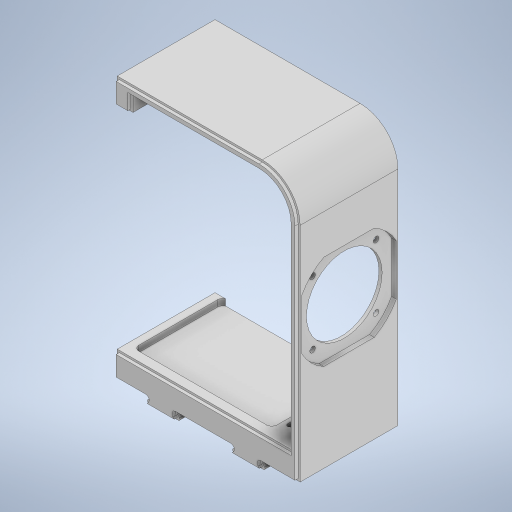
# Autodesk Inventor part: ElecTweetBox
Saved by Autodesk Inventor 2023 (Build 270158000, 158)
## iProperties
Created: 2022-07-12
Part Number: ElecTweetBox
Material: Generic
Document SubType Name: Modeling
Designer: Fuzzyfish
Density: 1 g/cm^3
Appearance: Default
Author: Fuzzyfish
Autodesk Inventor part; units mm, degrees
ref_plane "YZ Plane" through (0, 0, 0) normal (1, 0, 0) x (0, 1, 0)
ref_plane "XZ Plane" through (0, 0, 0) normal (0, 1, 0) x (-1, 0, 0)
ref_plane "XY Plane" through (0, 0, 0) normal (0, 0, 1) x (1, 0, 0)
sketch "Sketch1" plane through (0, 0, 0) normal (0, 0, 1) x (1, 0, 0)
  line L0 (0, 0) -> (116, 0)
  line L1 (116, 0) -> (116, 141)
  arc A0 (116, 141) -> (92, 165) centre (92, 141) ccw
  line L2 (0, 0) -> (0, 165)
  line L3 (0, 165) -> (92, 165)
  dimension "d0" = 24
  dimension "d1" = 92
  dimension "d2" = 165
  constraints: 8 end point, 2 horizontal, 2 point on circle, 2 tangent, 1 centre point, 1 perpendicular, 1 vertical
  measures "d0" radius of A0
  measures "d1" distance of L2.end L3.end
  measures "d2" distance of L0.start L2.end
extrude "Extrusion1" add sketch "Sketch1" along normal blind 62
shell "Shell2" thickness 5 removed faces 3 at (0, 110, 20.6667) at (38.6667, 102, 0) at (38.6667, 102, 62)
sketch "Sketch6" plane through (0, 160, 0) normal (0, -1, 0) x (1, 0, 0)
  line L0 (0, 0) -> (10, 0)
  line L1 (10, 0) -> (10, 10)
  line L2 (10, 10) -> (0, 10)
  line L3 (0, 10) -> (0, 0)
  dimension "d90" = 2
  dimension "d91" = 0
  dimension "d38" = 10
  dimension "d39" = 10
  constraints: 8 end point, 2 parallel, 1 horizontal, 1 perpendicular
  measures "d38" distance of L1.end L2.end
  measures "d39" distance of L0.end L1.end
sketch "Sketch7" plane through (0, 160, 0) normal (0, -1, 0) x (1, 0, 0)
  line L0 (0, 62) -> (10, 62)
  line L1 (10, 62) -> (10, 52)
  line L2 (10, 52) -> (0, 52)
  line L3 (0, 52) -> (0, 62)
  line L4 (92, 0) -> (0, 0) projected
  line L5 (92, 0) -> (92, 62) projected
  line L6 (0, 62) -> (92, 62) projected
  line L7 (0, 0) -> (0, 62) projected
  point P0 (0, 0)
  dimension "d40" = 10
  dimension "d41" = 10
  constraints: 8 end point, 2 parallel, 1 horizontal, 1 perpendicular
  measures "d40" distance of L1.end L2.end
  measures "d41" distance of L0.end L1.end
extrude "Extrusion6" add sketch "Sketch6" along normal blind 10
extrude "Extrusion7" add sketch "Sketch7" along normal blind 10 contours L0 L1 L2 L3
sketch "Sketch9" plane through (0, 5, 0) normal (0, 1, 0) x (1, 0, 0)
  line L0 (0, 0) -> (111, 0) projected
  line L1 (0, -62) -> (0, 0) projected
  line L2 (111, -62) -> (0, -62) projected
  line L3 (111, 0) -> (111, -62) projected
extrude "Extrusion8" add sketch "Sketch9" along normal blind 10
sketch "Sketch10" plane through (0, 15, 0) normal (0, 1, 0) x (1, 0, 0)
  arc A0 (5, -53) -> (8, -56) centre (8, -53) ccw
  arc A1 (8, 0) -> (5, -3) centre (8, -3) ccw
  line L0 (5, -53) -> (5, -3)
  arc A2 (92, -3) -> (89, 0) centre (89, -3) ccw
  arc A3 (89, -56) -> (92, -53) centre (89, -53) ccw
  line L1 (89, -56) -> (8, -56)
  line L2 (89, 0) -> (8, 0)
  line L3 (92, -53) -> (92, -3)
  line L4 (0, 0) -> (0, -62) projected
  line L5 (111, 0) -> (0, 0) projected
  arc A4 (4.7, -53) -> (8, -56.3) centre (8, -53) ccw
  line L6 (4.7, -53) -> (4.7, -3)
  arc A5 (8, 0.3) -> (4.7, -3) centre (8, -3) ccw
  line L7 (8, 0.3) -> (89, 0.3)
  arc A6 (92.3, -3) -> (89, 0.3) centre (89, -3) ccw
  line L8 (92.3, -3) -> (92.3, -53)
  arc A7 (89, -56.3) -> (92.3, -53) centre (89, -53) ccw
  line L9 (89, -56.3) -> (8, -56.3)
  point P0 (6.6252, 0)
  point P1 (90.3748, 0)
  point P2 (89, 0)
  dimension "d48" = 81
  dimension "d49" = 3
  dimension "d50" = 50
  dimension "d51" = 3
  dimension "d52" = 81
  dimension "d53" = 3
  dimension "d54" = 50
  dimension "d55" = 3
  dimension "d56" = 5
  dimension "d57" = 0.3
  constraints: 16 end point, 16 point on circle, 8 centre point, 6 tangent, 2 horizontal, 1 collinear, 1 vertical, 7 other
  measures "d48" distance of L1.start L1.end
  measures "d49" radius of A0
  measures "d50" distance of L0.start L0.end
  measures "d51" radius of A1
  measures "d52" distance of L2.start L2.end
  measures "d53" radius of A2
  measures "d54" distance of L3.start L3.end
  measures "d55" radius of A3
  measures "d56" distance between parallel lines of L0 L4
  measures "d57" distance between parallel lines of L9 L1
extrude "Extrusion9" cut sketch "Sketch10" against normal blind 4 contours L0 A1 L2 A2 L3 A3 L1 A0 | A0 L1 A3 L3 A2 L5 A6 L8 A7 L9 A4 L6 A5 A1 L0
sketch "Sketch12" plane through (0, 160, 10) normal (0, 0, 1) x (1, 0, 0)
  line L0 (0, 0) -> (10, 0) projected
  line L1 (0, 0) -> (0, -10) projected
  line L2 (10, -10) -> (0, -10) projected
  line L3 (10, 0) -> (10, -10) projected
  point P0 (0, -160)
extrude "Extrusion11" add sketch "Sketch12" along normal up to surface (42 mm away)
sketch "Sketch14" plane through (0, 0, 62) normal (0, 0, 1) x (1, 0, 0)
  line L0 (36.5757, 0) -> (41.5757, -5)
  line L1 (22, 0) -> (37, 0)
  line L2 (17.3, -4.7) -> (41.7, -4.7)
  line L3 (22.4243, 0) -> (17.4243, -5)
  line L4 (22, 0) -> (17, -5)
  line L5 (-3, 0) -> (-3, -5)
  line L6 (96, -5) -> (91, 0)
  line L7 (42, -5) -> (37, 0)
  line L8 (71, -5) -> (76, 0)
  line L9 (76.4243, 0) -> (71.4243, -5)
  line L10 (76, 0) -> (91, 0)
  line L11 (71.3, -4.7) -> (95.7, -4.7)
  line L12 (116, 0) -> (-3, 0)
  line L13 (-3, 0) -> (116, 0)
  line L14 (-3, -5) -> (116, -5)
  line L15 (90.5757, 0) -> (95.5757, -5)
  line L16 (116, 0) -> (116, -5)
  line L17 (10, 160) -> (92, 160) projected
  arc A0 (111, 141) -> (92, 160) centre (92, 141) ccw projected
  line L18 (111, 141) -> (111, 15) projected
  line L19 (0, 15) -> (111, 15) projected
  line L20 (0, 15) -> (0, 0) projected
  line L21 (0, 0) -> (116, 0) projected
  line L22 (116, 0) -> (116, 141) projected
  arc A1 (116, 141) -> (92, 165) centre (92, 141) ccw projected
  line L23 (92, 165) -> (0, 165) projected
  line L24 (0, 165) -> (0, 150) projected
  line L25 (10, 150) -> (0, 150) projected
  line L26 (10, 160) -> (10, 150) projected
  point P0 (95.2757, -4.7)
  point P1 (71.7243, -4.7)
  point P2 (17.7243, -4.7)
  point P3 (41.2757, -4.7)
  dimension "d70" = 5
  dimension "d71" = 45
  dimension "d72" = 45
  dimension "d73" = 45
  dimension "d74" = 20
  dimension "d75" = 25
  dimension "d76" = 25
  dimension "d77" = 20
  dimension "d78" = 119
  dimension "d79" = 0.3
  dimension "d80" = 0.3
  dimension "d81" = 0.3
  dimension "d82" = 0.3
  dimension "d83" = 0.3
  dimension "d84" = 0.3
  constraints: 32 end point, 12 point on line, 6 parallel, 2 collinear, 2 horizontal, 1 vertical, 11 other
  measures "d71" angle to the sketch x axis of L4
  measures "d72" angle to the sketch x axis of L7
  measures "d73" angle to the sketch x axis of L8
  measures "d74" distance of L5.end L4.end
  measures "d75" distance of L6.start L8.start
  measures "d76" distance of L4.end L7.start
  measures "d77" distance of L16.end L6.start
  measures "d78" distance between parallel lines of L16 L5
  measures "d79" distance between parallel lines of L4 L3
  measures "d80" distance between parallel lines of L7 L0
  measures "d82" distance between parallel lines of L8 L9
  measures "d84" distance between parallel lines of L6 L15
extrude "Extrusion12" add sketch "Sketch14" against normal up to surface (62 mm away) contours L0 L2 L3 L1 | L10 L15 L11 L9
fillet "Fillet4" radius 1 8 edges at (22.4243, 0, 31) (17.7243, -4.7, 31) (41.2757, -4.7, 31) (76.4243, 0, 31) (71.7243, -4.7, 31) (95.2757, -4.7, 31) (36.5757, 0, 31) (90.5757, 0, 31)
sketch "Sketch15" plane through (0, 0, 62) normal (0, 0, 1) x (1, 0, 0)
  arc A0 (92.8615, -4.7) -> (93.5686, -2.9929) centre (92.8615, -3.7) ccw projected
  line L0 (93.5686, -2.9929) -> (92.2828, -1.7071) projected
  arc A1 (92.9899, 0) -> (92.2828, -1.7071) centre (92.9899, -1) ccw projected
  line L1 (92.9899, 0) -> (116, 0) projected
  line L2 (116, 0) -> (116, 141) projected
  arc A2 (116, 141) -> (92, 165) centre (92, 141) ccw projected
  line L3 (92, 165) -> (0, 165) projected
  line L4 (0, 165) -> (0, 150) projected
  line L5 (10, 150) -> (0, 150) projected
  line L6 (10, 160) -> (10, 150) projected
  line L7 (10, 160) -> (92, 160) projected
  arc A3 (111, 141) -> (92, 160) centre (92, 141) ccw projected
  line L8 (111, 141) -> (111, 15) projected
  line L9 (0, 15) -> (111, 15) projected
  line L10 (0, 15) -> (0, 0) projected
  line L11 (0, 0) -> (20.0101, 0) projected
  arc A4 (20.7172, -1.7071) -> (20.0101, 0) centre (20.0101, -1) ccw projected
  line L12 (20.7172, -1.7071) -> (19.4314, -2.9929) projected
  arc A5 (19.4314, -2.9929) -> (20.1385, -4.7) centre (20.1385, -3.7) ccw projected
  line L13 (20.1385, -4.7) -> (38.8615, -4.7) projected
  arc A6 (38.8615, -4.7) -> (39.5686, -2.9929) centre (38.8615, -3.7) ccw projected
  line L14 (39.5686, -2.9929) -> (38.2828, -1.7071) projected
  arc A7 (38.9899, 0) -> (38.2828, -1.7071) centre (38.9899, -1) ccw projected
  line L15 (38.9899, 0) -> (74.0101, 0) projected
  arc A8 (74.7172, -1.7071) -> (74.0101, 0) centre (74.0101, -1) ccw projected
  line L16 (74.7172, -1.7071) -> (73.4314, -2.9929) projected
  arc A9 (73.4314, -2.9929) -> (74.1385, -4.7) centre (74.1385, -3.7) ccw projected
  line L17 (74.1385, -4.7) -> (92.8615, -4.7) projected
  line L18 (112.3, 13.7) -> (112.3, 141)
  arc A10 (112.3, 141) -> (92, 161.3) centre (92, 141) ccw
  line L19 (92, 161.3) -> (8.7, 161.3)
  line L20 (8.7, 161.3) -> (8.7, 151.3)
  line L21 (8.7, 151.3) -> (1.3, 151.3)
  line L22 (1.3, 151.3) -> (1.3, 163.7)
  line L23 (1.3, 163.7) -> (92, 163.7)
  arc A11 (114.7, 141) -> (92, 163.7) centre (92, 141) ccw
  line L24 (114.7, 141) -> (114.7, 1.3)
  line L25 (114.7, 1.3) -> (92.9899, 1.3)
  arc A12 (92.9899, 1.3) -> (91.3636, -2.6263) centre (92.9899, -1) ccw
  line L26 (91.3636, -2.6263) -> (92.1373, -3.4)
  line L27 (92.1373, -3.4) -> (74.8627, -3.4)
  line L28 (74.8627, -3.4) -> (75.6364, -2.6263)
  arc A13 (75.6364, -2.6263) -> (74.0101, 1.3) centre (74.0101, -1) ccw
  line L29 (74.0101, 1.3) -> (38.9899, 1.3)
  arc A14 (38.9899, 1.3) -> (37.3636, -2.6263) centre (38.9899, -1) ccw
  line L30 (37.3636, -2.6263) -> (38.1373, -3.4)
  line L31 (38.1373, -3.4) -> (20.8627, -3.4)
  line L32 (20.8627, -3.4) -> (21.6364, -2.6263)
  arc A15 (21.6364, -2.6263) -> (20.0101, 1.3) centre (20.0101, -1) ccw
  line L33 (20.0101, 1.3) -> (1.3, 1.3)
  line L34 (1.3, 1.3) -> (1.3, 13.7)
  line L35 (1.3, 13.7) -> (112.3, 13.7)
  dimension "d89" = 1.3
  constraints: 36 end point, 12 point on circle, 6 centre point, 23 other
  measures "d89" distance between parallel lines of L9 L35
extrude "Extrusion13" add sketch "Sketch15" along normal blind 2 contours L18 A10 L19 L20 L21 L22 L23 A11 L24 L25 A12 L26 L27 L28 A13 L29 A14 L30 L31 L32 A15 L33 L34 L35
sketch "Sketch16" plane through (0, 15, 0) normal (0, 1, 0) x (1, 0, 0)
  line L0 (96.5, -31) -> (96.5, -49) construction
  line L1 (95, -31) -> (95, -49)
  line L2 (98, -49) -> (98, -31)
  arc A0 (98, -31) -> (95, -31) centre (96.5, -31) ccw
  arc A1 (95, -49) -> (98, -49) centre (96.5, -49) ccw
  line L3 (92.3, -3) -> (92.3, -53) projected
  line L4 (0, -62) -> (111, -62) projected
  line L5 (116, 0) -> (116, -62) projected
  line L6 (116, 0) -> (116, -62) projected
  point P0 (0, 0)
  point P1 (96.5, -40)
  point P2 (116, -31)
  dimension "d92" = 18
  dimension "d93" = 3
  dimension "d95" = 13
  dimension "d98" = 18
  constraints: 8 end point, 4 point on circle, 4 tangent, 2 centre point, 2 midpoint, 1 parallel, 1 vertical
  measures "d92" distance of L0.start L0.end
  measures "d93" distance between parallel lines of L1 L2
  measures "d95" distance from line of L4 L0.end
  measures "d98" distance from line of L2 point (116, -31)
extrude "Extrusion14" cut sketch "Sketch16" against normal through all
sketch "Sketch17" plane through (116, 0, 0) normal (1, 0, 0) x (0, 0, -1)
  circle A0 centre (-51.1525, 65.8475) radius 1.8
  arc A1 (-61, 70) -> (-47, 56) centre (-31, 86) ccw
  line L0 (4, 51) -> (-66, 51)
  line L1 (-61, 56) -> (-1, 56) construction
  line L2 (-15, 56) -> (-47, 56)
  circle A2 centre (-10.8475, 65.8475) radius 1.8
  arc A3 (-15, 56) -> (-1, 70) centre (-31, 86) ccw
  line L3 (-1, 102) -> (-1, 70)
  circle A4 centre (-10.8475, 106.1525) radius 4 construction
  circle A5 centre (-10.8475, 106.1525) radius 1.8
  arc A6 (-1, 102) -> (-15, 116) centre (-31, 86) ccw
  line L4 (-61, 70) -> (-61, 102)
  line L5 (-61, 116) -> (-61, 56) construction
  arc A7 (-47, 116) -> (-61, 102) centre (-31, 86) ccw
  line L6 (-66, 51) -> (-66, 121)
  line L7 (-47, 116) -> (-15, 116)
  circle A8 centre (-31, 86) radius 23.5 construction
  circle A9 centre (-31, 86) radius 24
  line L8 (-1, 116) -> (-61, 56) construction
  line L9 (-61, 116) -> (-1, 56) construction
  line L10 (-1, 56) -> (-1, 116) construction
  line L11 (4, 121) -> (4, 51)
  circle A10 centre (-31, 86) radius 34 construction
  line L12 (4, 121) -> (-66, 51) construction
  line L13 (-66, 121) -> (4, 51) construction
  line L14 (-1, 116) -> (-61, 116) construction
  line L15 (-66, 121) -> (4, 121)
  circle A11 centre (-51.1525, 106.1525) radius 1.8
  line L16 (0, 0) -> (0, 141) projected
  line L17 (0, 141) -> (-62, 141) projected
  point P0 (-1, 102)
  point P1 (-47, 56)
  point P2 (-1, 70)
  point P3 (-15, 116)
  dimension "d101" = 60
  dimension "d102" = 60
  dimension "d103" = 68
  dimension "d104" = 47
  dimension "d105" = 8
  dimension "d106" = 28.5
  dimension "d107" = 3.6
  dimension "d108" = 48
  dimension "d109" = 360
  dimension "d110" = 70
  dimension "d111" = 70
  dimension "d114" = 20
  dimension "d119" = 1
  constraints: 32 end point, 12 centre point, 12 point on circle, 6 coincident, 4 midpoint, 4 parallel, 4 point on line, 2 horizontal, 2 perpendicular, 1 collinear, 1 concentric, 34 other
  measures "d101" distance of L10.start L10.end
  measures "d102" distance of L1.start L10.start
  measures "d103" diameter of A10
  measures "d104" diameter of A8
  measures "d105" diameter of A4
  measures "d106" distance of A4.centre point (-31, 86)
  measures "d107" diameter of A5
  measures "d108" diameter of A9
  measures "d110" distance of L11.start L11.end
  measures "d111" distance of L13.start L11.start
  measures "d114" distance between parallel lines of L17 L15
  measures "d119" distance of the line from the sketch origin of L10
extrude "Extrusion15" cut sketch "Sketch17" against normal blind 3 contours L4 A7 L7 A6 L3 A3 L2 A1
extrude "Extrusion16" cut sketch "Sketch17" against normal through all contours A0 | A2 | A5 | A9 | A11
sketch "Sketch18" plane through (0, 0, 0) normal (0, 0, -1) x (-1, 0, 0)
  circle A0 centre (-5, 153) radius 1.8
  line L0 (0, 150) -> (-10, 150) projected
  line L1 (-10, 160) -> (-10, 150) projected
  circle A1 centre (-111, 4) radius 1.8
  circle A2 centre (-5, 4) radius 1.8
  line L2 (-6.6252, 15) -> (0, 15) projected
  line L3 (0, 0) -> (-20.0101, 0) projected
  line L4 (-92.9899, 0) -> (-116, 0) projected
  line L5 (-116, 0) -> (-116, 141) projected
  line L6 (0, 15) -> (0, 0) projected
  dimension "d120" = 3.6
  dimension "d121" = 3
  dimension "d122" = 5
  dimension "d123" = 10
  dimension "d124" = 3.6
  dimension "d125" = 3.6
  dimension "d126" = 15
  dimension "d127" = 4
  dimension "d128" = 4
  dimension "d129" = 5
  dimension "d130" = 5
  constraints: 3 centre point
  measures "d120" diameter of A0
  measures "d121" distance from line of A0.centre L0
  measures "d122" distance from line of L1 A0.centre
  measures "d123" distance of L0.start L0.end
  measures "d124" diameter of A2
  measures "d125" diameter of A1
  measures "d126" distance between parallel lines of L2 L3
  measures "d127" distance from line of L3 A2.centre
  measures "d128" distance from line of L4 A1.centre
  measures "d129" distance from line of L5 A1.centre
  measures "d130" distance from line of L6 A2.centre
extrude "Extrusion17" cut sketch "Sketch18" against normal blind 10
sketch "Sketch19" plane through (0, 165, 0) normal (-1, 0, 0) x (0, 0, 1)
  line L0 (10, -13.8) -> (10, -10.2) projected
  line L1 (0, -13.8) -> (0, -10.2) projected
  circle A0 centre (5, -5) radius 1.8
  circle A1 centre (57, -5) radius 1.8
  circle A2 centre (5, -156.5) radius 1.8
  circle A3 centre (57, -156.5) radius 1.8
  line L2 (0, -5) -> (62.0541, -5) construction
  line L3 (0, 0) -> (62, 0) construction
  line L4 (62, 0) -> (62, -15) construction
  line L5 (0, 0) -> (0, -15) construction
  line L6 (62, -150) -> (62, -165) construction
  line L7 (0, -150) -> (62, -150) construction
  line L8 (0, -150) -> (0, -165) construction
  dimension "d133" = 3.6
  dimension "d134" = 3.6
  dimension "d135" = 3.6
  dimension "d136" = 3.6
  dimension "d137" = 5
  dimension "d138" = 5
  dimension "d139" = 5
  dimension "d140" = 5
  dimension "d141" = 5
  dimension "d142" = 6.5
  dimension "d143" = 5
  dimension "d144" = 6.5
  constraints: 4 centre point, 2 end point, 1 horizontal, 1 point on line
  measures "d133" diameter of A0
  measures "d134" diameter of A2
  measures "d135" diameter of A3
  measures "d136" diameter of A1
  measures "d137" distance from line of L3 A0.centre
  measures "d138" distance from line of L3 A1.centre
  measures "d139" distance from line of L4 A1.centre
  measures "d140" distance from line of L5 A0.centre
  measures "d141" distance from line of L6 A3.centre
  measures "d142" distance from line of L7 A3.centre
  measures "d143" distance from line of L8 A2.centre
  measures "d144" distance from line of L7 A2.centre
extrude "Extrusion18" cut sketch "Sketch19" against normal blind 10
body "Solid1"
